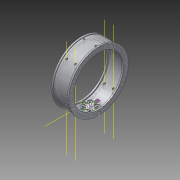
# Autodesk Inventor part: Rotorkopf
Saved by Autodesk Inventor 2013 (Build 170138000, 138)
## iProperties
Created: 2012-12-21
Part Number: Rotorkopf
Material: Aluminium 6061
Document SubType Name: Modeling
Designer: Lukas
Density: 1 g/cm^3
Author: Lukas
Autodesk Inventor part; units mm, degrees
note: some values were not read from the file. Chosen so that the rebuilt part matches the saved one: direction of "Bohrung9".
sketch "Skizze1" plane through (0, 0, 0) normal (1, 0, 0) x (0, 1, 0)
  circle A0 centre (0, 0) radius 102.5
  dimension "d0" = 205
  constraints: 1 centre point, 1 coincident
  measures "d0" diameter of A0
extrude "Extrusion1" add sketch "Skizze1" along normal blind 5
sketch "Skizze2" plane through (5, 0, 0) normal (1, 0, 0) x (0, 0, -1)
  circle A0 centre (0, 0) radius 102.5 projected
  circle A1 centre (0, 0) radius 100
  dimension "d3" = 200
  constraints: 1 centre point, 1 coincident
  measures "d3" diameter of A1
extrude "Extrusion2" add sketch "Skizze2" along normal blind 50 contours A1
sketch "Skizze3" plane through (55, 0, 0) normal (1, 0, 0) x (0, 0, -1)
  circle A0 centre (0, 0) radius 100 projected
  circle A1 centre (0, 0) radius 102.5
  dimension "d6" = 205
  constraints: 1 centre point, 1 coincident
  measures "d6" diameter of A1
extrude "Extrusion3" add sketch "Skizze3" along normal blind 5 contours A0 | A1
sketch "Skizze7" plane through (0, 0, 0) normal (-1, 0, 0) x (0, 0, 1)
  circle A0 centre (0, 0) radius 102.5 projected
  circle A1 centre (0, 0) radius 90
  dimension "d17" = 180
  constraints: 1 centre point, 1 coincident
  measures "d17" diameter of A1
extrude "Extrusion6" cut sketch "Skizze7" against normal blind 60 contours A1
sketch "Skizze8" plane through (0, 0, 0) normal (-1, 0, 0) x (0, 0, 1)
  circle A0 centre (0, 0) radius 90 projected
  circle A1 centre (0, 0) radius 102.5 projected
  circle A2 centre (0, 0) radius 90
  circle A3 centre (0, 0) radius 85
  dimension "d20" = 170
  constraints: 2 centre point, 2 coincident, 1 concentric
  measures "d20" diameter of A3
extrude "Extrusion7" add sketch "Skizze8" against normal blind 5 contours A0
sketch "Skizze9" plane through (60, 0, 0) normal (1, 0, 0) x (0, 0, -1)
  circle A0 centre (0, 0) radius 90 projected
  circle A1 centre (0, 0) radius 102.5 projected
  circle A2 centre (0, 0) radius 90
  circle A3 centre (0, 0) radius 85
  dimension "d23" = 170
  constraints: 2 centre point, 2 coincident, 1 concentric
  measures "d23" diameter of A3
extrude "Extrusion8" add sketch "Skizze9" against normal blind 5 contours A0
sketch "Skizze22" plane through (60, 0, 0) normal (1, 0, 0) x (0, 0, -1)
  circle A0 centre (0, 0) radius 102.5 projected
  line L0 (89.5, 0) -> (89.5, 5)
  line L1 (89.5, 5) -> (102.378, 5)
  line L2 (89.5, 0) -> (89.5, -5)
  line L3 (89.5, -5) -> (102.378, -5)
  arc A1 (102.378, -5) -> (102.378, 5) centre (0, 0) ccw
  dimension "d186" = 5
  dimension "d187" = 90
  dimension "d188" = 5
  dimension "d203" = 13
  constraints: 8 end point, 4 point on circle, 2 perpendicular, 1 centre point, 1 coincident, 1 vertical
  measures "d186" distance of L0.start L0.end
  measures "d187" angle of L0 L1
  measures "d188" distance of L0.start L2.end
  measures "d203" distance edge to line of A0 L2
extrude "Extrusion14" cut sketch "Skizze22" against normal blind 60 contours A0 L3 L2 L0 L1 picked at (93.8153, -2.778)
ref_plane "Arbeitsebene4" through (0, 0, -102.5) normal (0, 0, -1) x (-1, 0, 0)
sketch "Skizze23" plane through (0, 0, -102.5) normal (0, 0, -1) x (-1, 0, 0)
  circle A0 centre (-30, 0) radius 30
  point P0 (0, 0)
  dimension "d191" = 60
  constraints: 1 centre point, 1 coincident
  measures "d191" diameter of A0
hole "Bohrung6" at (30, 0, -102.5) direction (0, 0, 1) diameter 60 depth 8
sketch "Skizze24" plane through (30, 0, -94.5) normal (0, 0, -1) x (-1, 0, 0)
  line L0 (29.5804, 5) -> (-29.5804, 5) projected
  arc A0 (29.5804, 5) -> (-29.5804, 5) centre (0, 0) ccw projected
  line L1 (0, 0) -> (5, 0)
  line L2 (5, 0) -> (5, 29.5804)
  line L3 (0, 0) -> (-5, 0)
  line L4 (-5, 0) -> (-5, 29.5804)
  line L5 (5, 0) -> (5, -29.6518)
  line L6 (-5, 0) -> (-5, -29.6518)
  arc A1 (5, 29.5804) -> (-5, 29.5804) centre (0, 0) ccw
  arc A2 (-5, -29.6518) -> (5, -29.6518) centre (0, 0) ccw
  point P0 (30, 0)
  dimension "d199" = 5
  dimension "d200" = 5
  constraints: 12 end point, 6 point on circle, 3 parallel, 2 centre point, 2 coincident, 2 perpendicular, 1 concentric
  measures "d199" distance of L1.start L1.end
  measures "d200" distance of L1.start L3.end
extrude "Extrusion15" cut sketch "Skizze24" against normal blind 10 contours L2 L1 L3 L4 L0 | L0 L4 A0 L2 | L5 A2 L6 L3 L1
sketch "Skizze26" plane through (60, -5, -89.5) normal (0, 0, -1) x (-1, 0, 0)
  arc A0 (35, 34.5804) -> (25, 34.5804) centre (30, 5) ccw projected
  point P0 (60, 5)
  point P1 (30, 23)
  point P2 (48, 5)
  point P3 (30, -13)
  point P4 (12, 5)
  dimension "d224" = 18
  dimension "d225" = 18
  dimension "d226" = 18
  dimension "d227" = 18
  measures "d224" distance of A0.centre point (12, 5)
  measures "d225" distance of point (30, 23) A0.centre
  measures "d226" distance of A0.centre point (48, 5)
  measures "d227" distance of A0.centre point (30, -13)
sketch "Skizze27" plane through (59.5804, -5, -94.5) normal (0, 0, -1) x (-1, 0, 0)
  arc A0 (0, 0) -> (24.5804, -24.5804) centre (29.5804, 5) ccw projected
  circle A1 centre (29.5804, 5) radius 18
  line L0 (29.5804, 5) -> (42.3083, -7.7279)
  line L1 (29.5804, 5) -> (47.5804, 5) construction
  line L2 (29.5804, 5) -> (42.3083, 17.7279)
  line L3 (29.5804, 5) -> (16.8525, 17.7279)
  line L4 (29.5804, 5) -> (16.8525, -7.7279)
  point P0 (59.5804, 5)
  point P1 (42.3083, -7.7279)
  point P2 (16.8525, -7.7279)
  dimension "d235" = 36
  dimension "d236" = 45
  constraints: 10 end point, 6 point on circle, 3 coincident, 3 perpendicular, 1 centre point, 1 equal length, 1 horizontal
  measures "d235" diameter of A1
  measures "d236" angle of L0 L1
hole "Bohrung9" at (42.7279, 12.7279, -94.5) at (17.2721, 12.7279, -94.5) at (17.2721, -12.7279, -94.5) at (42.7279, -12.7279, -94.5) direction (0, 0, 1) diameter 5 end up to surface
ref_plane "Arbeitsebene6" through (60, 0, -85) normal (0, 0, -1) x (-1, 0, 0)
sketch "Skizze28" plane through (60, 0, -85) normal (0, 0, -1) x (-1, 0, 0)
  line L0 (30, 0) -> (42.7279, 12.7279)
  line L1 (30, 0) -> (48, 0) construction
  line L2 (30, 0) -> (42.7279, -12.7279)
  line L3 (30, 0) -> (17.2721, -12.7279)
  line L4 (30, 0) -> (17.2721, 12.7279)
  point P0 (60, 0)
  dimension "d245" = 45
  constraints: 10 end point, 4 coincident, 3 perpendicular, 1 equal length, 1 horizontal
  measures "d245" angle of L1 L0
hole "Bohrung10" at (42.7279, 12.7279, -85) at (17.2721, 12.7279, -85) at (17.2721, -12.7279, -85) at (42.7279, -12.7279, -85) direction (0, 0, -1) diameter 14 depth 6
ref_plane "Arbeitsebene7" through (5, 0, 100) normal (0, 0, 1) x (1, 0, 0)
sketch "Skizze30" plane through (5, 0, 100) normal (0, 0, 1) x (1, 0, 0)
  line L0 (-5, 102.5) -> (-5, -102.5) projected
  line L1 (55, -102.5) -> (55, 102.5) projected
  point P0 (-5, 0)
  point P1 (10, 65)
  point P2 (40, 65)
  point P3 (10, -65)
  point P4 (40, -65)
  point P5 (-5, -5)
  point P6 (-5, 5)
  point P7 (55, 5)
  point P8 (55, -5)
  dimension "d276" = 15
  dimension "d277" = 15
  dimension "d278" = 15
  dimension "d279" = 15
  measures "d276" distance from line of L0 point (10, -65)
  measures "d277" distance from line of L1 point (40, -65)
  measures "d278" distance from line of L1 point (40, 65)
  measures "d279" distance from line of L0 point (10, 65)
hole "Bohrung12" at (15, 65, 100) at (45, 65, 100) at (15, -65, 100) at (45, -65, 100) direction (0, 0, -1) diameter 5 end through all
thread "Gewinde44" size "M5x0.8" class "6H" standard "ANSI Metric M Profile" full length
thread "Gewinde45" size "M5x0.8" class "6H" standard "ANSI Metric M Profile" full length
thread "Gewinde46" size "M5x0.8" class "6H" standard "ANSI Metric M Profile" full length
thread "Gewinde47" size "M5x0.8" class "6H" standard "ANSI Metric M Profile" full length
thread "Gewinde48" size "M5x0.8" class "6H" standard "ANSI Metric M Profile" full length
thread "Gewinde49" size "M5x0.8" class "6H" standard "ANSI Metric M Profile" full length
thread "Gewinde50" size "M5x0.8" class "6H" standard "ANSI Metric M Profile" full length
thread "Gewinde51" size "M5x0.8" class "6H" standard "ANSI Metric M Profile" full length
thread "Gewinde52" size "M5x0.8" class "6H" standard "ANSI Metric M Profile" full length
thread "Gewinde53" size "M5x0.8" class "6H" standard "ANSI Metric M Profile" full length
thread "Gewinde54" size "M5x0.8" class "6H" standard "ANSI Metric M Profile" full length
thread "Gewinde55" size "M5x0.8" class "6H" standard "ANSI Metric M Profile" full length
sketch "Skizze31" plane through (5, 0, 100) normal (0, 0, 1) x (1, 0, 0)
  line L0 (55, -102.5) -> (55, 102.5) projected
  point P0 (-5, 0)
  point P1 (5, 0)
  point P2 (45, 0)
  point P3 (55, 5)
  point P4 (55, -5)
  dimension "d333" = 10
  dimension "d334" = 10
  measures "d333" distance of point (-5, 0) point (5, 0)
  measures "d334" distance from line of point (45, 0) L0
ref_plane "Arbeitsebene9" through (5, -100, 0) normal (0, -1, 0) x (1, 0, 0)
ref_plane "Arbeitsebene10" through (5, 100, 0) normal (0, 1, 0) x (-1, 0, 0)
sketch "Skizze32" plane through (5, 100, 0) normal (0, 1, 0) x (-1, 0, 0)
  line L0 (-55, 102.5) -> (-55, -102.378) projected
  line L1 (5, -102.378) -> (5, 102.5) projected
  point P0 (5, 0)
  point P1 (-5, 0)
  point P2 (-45, 0)
  dimension "d335" = 10
  dimension "d336" = 10
  measures "d335" distance from line of L0 point (-45, 0)
  measures "d336" distance from line of L1 point (-5, 0)
hole "Bohrung13" at (50, 100, 0) at (10, 100, 0) direction (0, -1, 0) diameter 5 end through all
hole "Bohrung14" at (10, 0, 100) at (50, 0, 100) direction (0, 0, -1) diameter 5 end through all
